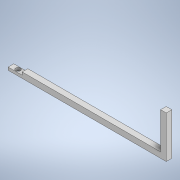
# Autodesk Inventor part: brace2
Saved by Autodesk Inventor 2020.2 (Build 242310000, 310)
## iProperties
Created: 2020-02-12
Part Number: brace2
Material: Generic
Document SubType Name: Modeling
Designer: ColinP
Density: 1 g/cm^3
Appearance: Default
Author: ColinP
Autodesk Inventor part; units mm, degrees
ref_plane "YZ Plane" through (0, 0, 0) normal (1, 0, 0) x (0, 1, 0)
ref_plane "XZ Plane" through (0, 0, 0) normal (0, 1, 0) x (-1, 0, 0)
ref_plane "XY Plane" through (0, 0, 0) normal (0, 0, 1) x (1, 0, 0)
sketch "Sketch1" plane through (0, 0, 0) normal (0, 1, 0) x (-1, 0, 0)
  line L0 (0, 0) -> (98.679, 0)
  line L1 (98.679, 0) -> (98.679, -4)
  line L2 (98.679, -4) -> (0, -4)
  line L3 (0, -4) -> (0, 0)
  line L4 (0, -4) -> (-4, -4)
  line L5 (-4, -4) -> (-4, 0)
  line L6 (-4, 0) -> (0, 0)
  line L7 (0, 0) -> (0, -4)
  line L8 (98.679, 0) -> (108.679, 0)
  line L9 (108.679, 0) -> (108.679, -4)
  line L10 (108.679, -4) -> (98.679, -4)
  dimension "d0" = 98.679
  dimension "d1" = 4
  dimension "d2" = 4
  dimension "d3" = 4
  dimension "d4" = 10
  constraints: 22 end point, 4 parallel, 3 horizontal, 3 perpendicular, 1 collinear
  measures "d0" distance of L1.end L2.end
  measures "d1" distance of L0.end L1.end
  measures "d2" distance of L5.end L6.end
  measures "d3" distance of L4.end L5.end
  measures "d4" distance of L0.end L8.end
extrude "Extrusion1" add sketch "Sketch1" along normal blind 30 contours L3 L4 L5 L6
extrude "Extrusion2" add sketch "Sketch1" along normal blind 4 contours L0 L1 L2 L3 | L8 L9 L10 L1
sketch "Sketch2" plane through (0, 4, 0) normal (0, 1, 0) x (1, 0, 0)
  line L0 (-108.679, 4) -> (-108.679, 0) projected
  line L1 (-108.679, 2) -> (-103.679, 2)
  point P0 (0, 0)
  dimension "d9" = 5
  constraints: 2 end point, 1 horizontal, 1 midpoint
  measures "d9" distance of L1.start L1.end
hole "Hole1" at (-103.679, 4, -2) direction (0, -1, 0) diameter 3.4 end through all clearance for "Flat Head Machine Screw" size "M3" standard "Ansi Metric M Profile"
sketch "Sketch3" plane through (-108.679, 0, -4) normal (-1, 0, 0) x (0, 0, 1)
  line L0 (0, 4) -> (4, 4) projected
  line L1 (0, 4) -> (4, 4)
  line L2 (4, 4) -> (4, 2)
  line L3 (4, 2) -> (0, 2)
  line L4 (0, 2) -> (0, 4)
  point P0 (4, 0)
  dimension "d17" = 4
  dimension "d18" = 2
  constraints: 8 end point, 2 parallel, 1 horizontal, 1 perpendicular
  measures "d17" distance of L2.end L3.end
  measures "d18" distance of L1.end L2.end
extrude "Extrusion3" cut sketch "Sketch3" against normal blind 10
body "Solid1"
